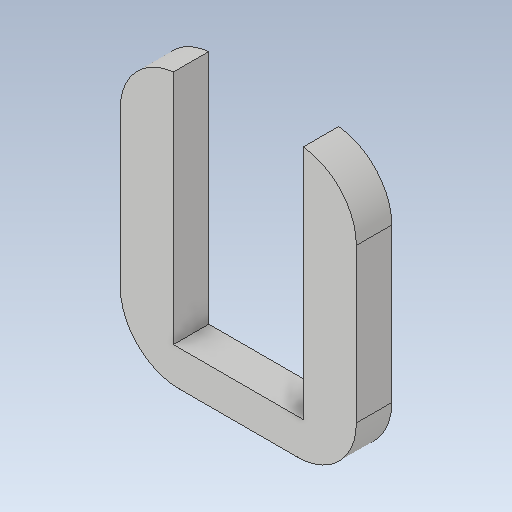
# Autodesk Inventor part: seguro2
Saved by Autodesk Inventor 2020 (Build 240168000, 168)
## iProperties
Created: 2020-01-12
Part Number: seguro2
Material: Generic
Document SubType Name: Modeling
Designer: Laptop
Density: 1 g/cm^3
Appearance: Default
Author: Laptop
Autodesk Inventor part; units mm, degrees
ref_plane "YZ Plane" through (0, 0, 0) normal (1, 0, 0) x (0, 1, 0)
ref_plane "XZ Plane" through (0, 0, 0) normal (0, 1, 0) x (-1, 0, 0)
ref_plane "XY Plane" through (0, 0, 0) normal (0, 0, 1) x (1, 0, 0)
sketch "Boceto1" plane through (0, 0, 0) normal (0, 0, 1) x (1, 0, 0)
  line L0 (-10, -10) -> (10, -10)
  line L1 (10, -10) -> (10, 10)
  line L2 (-10, 10) -> (-10, -10)
  line L3 (-10, -10) -> (10, 10) construction
  line L4 (10, -10) -> (-10, 10) construction
  circle A0 centre (0, 0) radius 5.5
  line L5 (-5.5, 0) -> (-5.5, 11.2745)
  line L6 (-5.5, 11.2745) -> (-5.5, 10)
  line L7 (5.5, 0) -> (5.5, 6.4261)
  line L8 (5.5, 6.4261) -> (5.5, 10.6373)
  line L9 (-5.5, 0) -> (-5.5, -7)
  line L10 (-5.5, -7) -> (5.5, -7)
  line L11 (5.5, -7) -> (5.5, 0)
  line L12 (-5.5, 10) -> (-5.5, 13)
  line L13 (-5.5, 13) -> (-10, 13)
  line L14 (-10, 13) -> (-10, 10)
  line L15 (5.5, 10) -> (5.5, 13)
  line L16 (10, 13) -> (10, 10)
  line L17 (5.5, 13) -> (10, 13)
  dimension "d0" = 20
  dimension "d1" = 20
  dimension "d2" = 11
  dimension "d4" = 7
  dimension "d5" = 3
  dimension "d6" = 23
  constraints: 36 end point, 7 point on line, 5 perpendicular, 4 vertical, 3 parallel, 3 tangent, 2 midpoint, 2 point on circle, 1 centre point, 1 coincident
  measures "d0" distance of L2.start L1.end
  measures "d1" distance of L1.end L0.end
  measures "d2" diameter of A0
  measures "d4" distance of L5.start L9.end
  measures "d5" distance of L6.end L12.end
extrude "Extrusión1" add sketch "Boceto1" along normal blind 3 contours L2 L14 L13 L12 L5 L9 L10 L11 L7 L8 L15 L17 L16 L1 L0
fillet "Empalme1" radius 5 4 edges at (10, -10, 1.5) (-10, -10, 1.5) (-10, 13, 1.5) (10, 13, 1.5)
